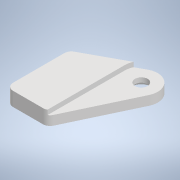
# Autodesk Inventor part: bonnet_fixator
Saved by Autodesk Inventor 2022 (Build 260153000, 153)
## iProperties
Created: 2025-03-29
Part Number: bonnet_fixator
Material: Типовые
Document SubType Name: Modeling
Designer: akap
Density: 1 g/cm^3
Appearance: По умолчанию
Author: akap
Autodesk Inventor part; units mm, degrees
ref_plane "YZ Plane" through (0, 0, 0) normal (1, 0, 0) x (0, 1, 0)
ref_plane "XZ Plane" through (0, 0, 0) normal (0, 1, 0) x (-1, 0, 0)
ref_plane "XY Plane" through (0, 0, 0) normal (0, 0, 1) x (1, 0, 0)
sketch "Эскиз1" plane through (0, 0, 0) normal (0, 1, 0) x (-1, 0, 0)
  circle A0 centre (0, 0) radius 1.35
  line L0 (0.5, -3.5) -> (-48.5, -3.5) projected
  arc A1 (-51.5, -0.5) -> (-48.5, -3.5) centre (-48.5, -0.5) ccw projected
  line L1 (-51.5, -0.5) -> (-51.5, 33.5) projected
  arc A2 (-48.5, 36.5) -> (-51.5, 33.5) centre (-48.5, 33.5) ccw projected
  line L2 (-48.5, 36.5) -> (0.5, 36.5) projected
  arc A3 (3.5, 33.5) -> (0.5, 36.5) centre (0.5, 33.5) ccw projected
  line L3 (3.5, 33.5) -> (3.5, -0.5) projected
  arc A4 (0.5, -3.5) -> (3.5, -0.5) centre (0.5, -0.5) ccw projected
  circle A5 centre (-48, 33) radius 1.35 projected
  circle A6 centre (0, 33) radius 1.35 projected
  circle A7 centre (-48, 0) radius 1.35 projected
  circle A8 centre (0, 0) radius 1.35 projected
  line L4 (-48.5, -3.8) -> (0.5, -3.8)
  arc A9 (0.5, -3.8) -> (3.8, -0.5) centre (0.5, -0.5) ccw
  line L5 (3.8, -0.5) -> (3.8, 33.5)
  arc A10 (3.8, 33.5) -> (0.5, 36.8) centre (0.5, 33.5) ccw
  line L6 (0.5, 36.8) -> (-48.5, 36.8)
  arc A11 (-48.5, 36.8) -> (-51.8, 33.5) centre (-48.5, 33.5) ccw
  line L7 (-51.8, 33.5) -> (-51.8, -0.5)
  arc A12 (-51.8, -0.5) -> (-48.5, -3.8) centre (-48.5, -0.5) ccw
  circle A13 centre (0, 0) radius 3.5
  line L8 (1.6675, -3.0773) -> (12.7, 2.901)
  line L9 (10.5, 14.101) -> (6, 14.101)
  line L10 (6, 14.101) -> (6, 5.101)
  line L11 (6, 5.101) -> (10.5, 5.101)
  line L12 (10.5, 5.101) -> (10.5, 14.101)
  line L13 (5.8, 4.901) -> (5.8, 14.301)
  line L14 (5.8, 14.301) -> (10.7, 14.301)
  line L15 (10.7, 14.301) -> (10.7, 4.901)
  line L16 (10.7, 4.901) -> (5.8, 4.901)
  line L17 (3.8, 2.901) -> (3.8, 16.301)
  line L18 (3.8, 16.301) -> (12.7, 16.301)
  line L19 (12.7, 16.301) -> (12.7, 2.901)
  line L20 (12.7, 2.901) -> (3.8, 2.901)
  line L21 (-3.1671, 1.4898) -> (3.8, 16.301)
  line L22 (19.4615, 18.801) -> (-3.6385, 18.801) projected
  dimension "d0" = 2.7
  dimension "d1" = 0.3
  dimension "d2" = 7
  dimension "d3" = 4.5
  dimension "d4" = 9
  dimension "d5" = 0.2
  dimension "d6" = 2
  dimension "d7" = 2.5
  constraints: 36 end point, 10 point on circle, 6 centre point, 6 parallel, 3 perpendicular, 2 coincident, 2 tangent, 1 horizontal, 1 point on line, 13 other
  measures "d0" diameter of A0
  measures "d1" distance between parallel lines of L0 L4
  measures "d2" diameter of A13
  measures "d3" distance of L11.end L10.end
  measures "d4" distance of L10.end L9.end
  measures "d5" distance between parallel lines of L10 L13
  measures "d6" distance between parallel lines of L16 L20
  measures "d7" distance between parallel lines of L18 L22
extrude "Выдавливание1" add sketch "Эскиз1" against normal blind 2 contours A13 | L8 A13 L3 A4 | A4 L3 L21 L5 A9 L8 | L21 L3 A13 | A9 L5 L20 L8 | L20 L5 L18 L19
chamfer "Фаска1" distance 1 angle 45 1 edges at (1.35, -2, 0)
fillet "Сопряжение1" radius 1.5 3 edges at (-12.7, -1, 2.901) (-3.8, -1, 16.301) (-12.7, -1, 16.301)
sketch "Эскиз2" plane through (0, 0, 0) normal (0, 1, 0) x (1, 0, 0)
  line L0 (-0.5, 3.5) -> (48.5, 3.5) projected
  arc A0 (51.5, 0.5) -> (48.5, 3.5) centre (48.5, 0.5) ccw projected
  line L1 (51.5, 0.5) -> (51.5, -33.5) projected
  arc A1 (48.5, -36.5) -> (51.5, -33.5) centre (48.5, -33.5) ccw projected
  line L2 (48.5, -36.5) -> (-0.5, -36.5) projected
  arc A2 (-3.5, -33.5) -> (-0.5, -36.5) centre (-0.5, -33.5) ccw projected
  line L3 (-3.5, -33.5) -> (-3.5, 0.5) projected
  arc A3 (-0.5, 3.5) -> (-3.5, 0.5) centre (-0.5, 0.5) ccw projected
  circle A4 centre (48, -33) radius 1.35 projected
  circle A5 centre (0, -33) radius 1.35 projected
  circle A6 centre (48, 0) radius 1.35 projected
  circle A7 centre (0, 0) radius 1.35 projected
  line L4 (48.5, 4) -> (-0.5, 4)
  arc A8 (-0.5, 4) -> (-4, 0.5) centre (-0.5, 0.5) ccw
  line L5 (-4, 0.5) -> (-4, -33.5)
  arc A9 (-4, -33.5) -> (-0.5, -37) centre (-0.5, -33.5) ccw
  line L6 (-0.5, -37) -> (48.5, -37)
  arc A10 (48.5, -37) -> (52, -33.5) centre (48.5, -33.5) ccw
  line L7 (52, -33.5) -> (52, 0.5)
  arc A11 (52, 0.5) -> (48.5, 4) centre (48.5, 0.5) ccw
  arc A12 (-12.7, -14.801) -> (-11.2, -16.301) centre (-11.2, -14.801) ccw projected
  line L8 (-11.2, -16.301) -> (-4.7521, -16.301) projected
  arc A13 (-4.7521, -16.301) -> (-3.3947, -15.4395) centre (-4.7521, -14.801) ccw projected
  line L9 (-3.3947, -15.4395) -> (3.1671, -1.4898) projected
  arc A14 (3.1671, -1.4898) -> (-1.6675, 3.0773) centre (0, 0) ccw projected
  line L10 (-1.6675, 3.0773) -> (-11.9146, -2.4754) projected
  arc A15 (-11.9146, -2.4754) -> (-12.7, -3.7943) centre (-11.2, -3.7943) ccw projected
  line L11 (-12.7, -3.7943) -> (-12.7, -14.801) projected
  circle A16 centre (0, 0) radius 1.35 projected
  line L12 (-5.8, -4.901) -> (-5.8, -14.301) projected
  line L13 (-5.8, -14.301) -> (-10.7, -14.301) projected
  line L14 (-10.7, -14.301) -> (-10.7, -4.901) projected
  line L15 (-10.7, -4.901) -> (-5.8, -4.901) projected
  point P0 (-4, -16.0988)
  point P1 (-3.6646, 1.9951)
  dimension "d6" = 2
  dimension "d14" = 0.5
  constraints: 8 end point, 8 point on circle, 4 centre point, 7 other
  measures "d14" distance between parallel lines of L0 L4
extrude "Выдавливание2" add sketch "Эскиз2" along normal blind 1 contours A8 L5 A13 L8 A12 L11 A15 L10 | L12 L13 L14 L15
